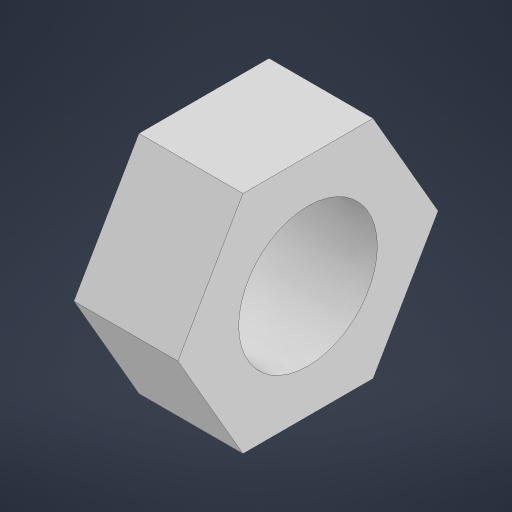
# Autodesk Inventor part: OcM8
Saved by Autodesk Inventor 2023 (Build 270158000, 158)
## iProperties
Created: 2023-09-09
Part Number: OcM8
Material: Generic
Document SubType Name: Modeling
Designer: philo
Density: 1 g/cm^3
Appearance: Default
Author: philo
Autodesk Inventor part; units mm, degrees
ref_plane "YZ Plane" through (0, 0, 0) normal (1, 0, 0) x (0, 1, 0)
ref_plane "XZ Plane" through (0, 0, 0) normal (0, 1, 0) x (-1, 0, 0)
ref_plane "XY Plane" through (0, 0, 0) normal (0, 0, 1) x (1, 0, 0)
sketch "Sketch1" plane through (0, 0, 0) normal (1, 0, 0) x (0, 1, 0)
  line L0 (6.5, -3.7528) -> (0, -7.5056)
  line L1 (0, -7.5056) -> (-6.5, -3.7528)
  line L2 (-6.5, -3.7528) -> (-6.5, 3.7528)
  line L3 (-6.5, 3.7528) -> (0, 7.5056)
  line L4 (0, 7.5056) -> (6.5, 3.7528)
  line L5 (6.5, 3.7528) -> (6.5, -3.7528)
  line L6 (0, 10.5078) -> (0, -10.5078) projected
  circle A0 centre (0, 0) radius 4
  dimension "d0" = 6.5
  dimension "d1" = 8
  constraints: 12 end point, 2 coincident, 1 centre point, 1 parallel, 13 other
  measures "d0" distance from line of L5 point (0, 0)
  measures "d1" diameter of A0
extrude "Extrusion1" add sketch "Sketch1" along normal blind 6 contours L0 L6 A0 L4 L5 | L1 L2 L3 L6 A0
body "Solid1"
